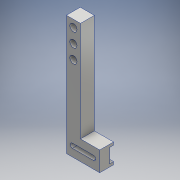
# Autodesk Inventor part: HeadbarHolder
Saved by Autodesk Inventor 2016 (Build 200138000, 138)
## iProperties
Created: 2015-11-10
Part Number: HeadbarHolder
Material: Aluminum 6061
Document SubType Name: Modeling
Designer: runeala
Density: 2.7 g/cm^3
Appearance: Aluminum - Flat
Mass: 44.5378 g
Surface Area: 80.2858 cm^2
Volume: 16.4955 cm^3
Author: runeala
Autodesk Inventor part; units mm, degrees
ref_plane "YZ Plane" through (0, 0, 0) normal (1, 0, 0) x (0, 1, 0)
ref_plane "XZ Plane" through (0, 0, 0) normal (0, 1, 0) x (-1, 0, 0)
ref_plane "XY Plane" through (0, 0, 0) normal (0, 0, 1) x (1, 0, 0)
sketch "Sketch1" plane through (0, 0, 0) normal (0, 1, 0) x (-1, 0, 0)
  line L0 (0, 0) -> (30, 0)
  line L1 (30, 0) -> (30, 108)
  line L2 (30, 108) -> (17.3, 108)
  line L3 (17.3, 108) -> (17.3, 17.8)
  line L4 (17.3, 17.8) -> (0, 17.8)
  line L5 (0, 17.8) -> (0, 0)
  dimension "d0" = 30
  dimension "d1" = 108
  dimension "d2" = 12.7
  dimension "d3" = 90.2
  constraints: 12 end point, 5 perpendicular, 1 horizontal
  measures "d0" distance of L0.start L0.end
  measures "d1" distance of L0.end L1.end
  measures "d2" distance of L1.end L2.end
  measures "d3" distance of L2.end L3.end
extrude "Extrusion1" add sketch "Sketch1" along normal blind 12.5
sketch "Sketch2" plane through (0, 12.5, 0) normal (0, 1, 0) x (1, 0, 0)
  line L0 (0, -17.8) -> (0, 0) projected
  line L1 (-30, 0) -> (-30, -108) projected
  line L2 (-30, 0) -> (-30, -108) projected
  line L3 (0, -15.3) -> (-30, -15.3)
  line L4 (-30, -15.3) -> (-30, -2.5)
  line L5 (-30, -2.5) -> (0, -2.5)
  line L6 (0, -2.5) -> (0, -15.3)
  dimension "d6" = 12.8
  constraints: 8 end point, 2 parallel, 2 point on line, 1 horizontal, 1 perpendicular
  measures "d6" distance of L3.end L4.end
extrude "Extrusion2" cut sketch "Sketch2" against normal blind 3.5
sketch "Sketch3" plane through (0, 9, 0) normal (0, 1, 0) x (1, 0, 0)
  line L0 (-30, -8.9) -> (0, -8.9) construction
  line L1 (0, -17.8) -> (0, 0) projected
  arc A0 (-5.5, -10.9) -> (-5.5, -6.9) centre (-5.5, -8.9) ccw
  arc A1 (-24.5, -6.9) -> (-24.5, -10.9) centre (-24.5, -8.9) ccw
  line L2 (-24.5, -10.9) -> (-5.5, -10.9)
  line L3 (-5.5, -6.9) -> (-24.5, -6.9)
  dimension "d9" = 4
  dimension "d10" = 4
  constraints: 6 end point, 4 point on circle, 2 centre point, 2 point on line, 1 horizontal, 1 midpoint, 1 parallel
  measures "d9" diameter of A0
  measures "d10" diameter of A1
extrude "Extrusion3" cut sketch "Sketch3" against normal through all
sketch "Sketch4" plane through (0, 12.5, 0) normal (0, 1, 0) x (1, 0, 0)
  line L0 (-30, -108) -> (-17.3, -108) projected
  line L1 (-23.65, -108) -> (-23.65, -15.5103) construction
  circle A0 centre (-23.65, -101.5) radius 5.5
  circle A1 centre (-23.65, -89) radius 5.5
  circle A2 centre (-23.65, -76.5) radius 5.5
  circle A3 centre (-23.65, -76.5) radius 3.25
  circle A4 centre (-23.65, -89) radius 3.25
  circle A5 centre (-23.65, -101.5) radius 3.25
  point P0 (0, 0)
  dimension "d13" = 11
  dimension "d14" = 11
  dimension "d15" = 11
  dimension "d16" = 12.5
  dimension "d17" = 12.5
  dimension "d18" = 6.5
  dimension "d19" = 6.5
  dimension "d20" = 6.5
  dimension "d25" = 6.5
  constraints: 6 centre point, 3 coincident, 3 point on line, 2 end point, 1 midpoint, 1 vertical
  measures "d13" diameter of A0
  measures "d14" diameter of A1
  measures "d15" diameter of A2
  measures "d16" distance of A1.centre A0.centre
  measures "d17" distance of A2.centre A1.centre
  measures "d18" diameter of A3
  measures "d19" diameter of A4
  measures "d20" diameter of A5
  measures "d25" distance from line of A0.centre L0
extrude "Extrusion4" cut sketch "Sketch4" against normal through all contours A3 | A4 | A5
extrude "Extrusion5" cut sketch "Sketch4" against normal blind 6
body "Solid1"
